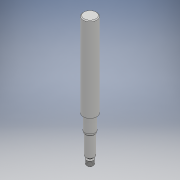
# Autodesk Inventor part: 도면1-2번
Saved by Autodesk Inventor 2018.3 (Build 223284000, 284)
## iProperties
Created: 2019-10-11
Part Number: 도면1-2번
Material: 일반
Document SubType Name: Modeling
Designer: MyTool
Density: 1 g/cm^3
Appearance: 기본값
Author: MyTool
Autodesk Inventor part; units mm, degrees
ref_plane "YZ Plane" through (0, 0, 0) normal (1, 0, 0) x (0, 1, 0)
ref_plane "XZ Plane" through (0, 0, 0) normal (0, 1, 0) x (-1, 0, 0)
ref_plane "XY Plane" through (0, 0, 0) normal (0, 0, 1) x (1, 0, 0)
sketch "스케치1" plane through (0, 0, 0) normal (1, 0, 0) x (0, 1, 0)
  line L0 (0, 0) -> (4, 0)
  line L1 (4, 0) -> (4, 10)
  line L2 (4, 10) -> (0, 10)
  line L3 (0, 10) -> (0, 0)
  line L4 (0, 10) -> (5, 10)
  line L5 (5, 10) -> (5, 33)
  line L6 (5, 33) -> (0, 33)
  line L7 (0, 33) -> (0, 10)
  line L8 (0, 33) -> (6, 33)
  line L9 (6, 33) -> (6, 53)
  line L10 (6, 53) -> (0, 53)
  line L11 (0, 53) -> (0, 33)
  line L12 (0, 53) -> (8, 53)
  line L13 (8, 53) -> (8, 153)
  line L14 (8, 153) -> (0, 153)
  line L15 (0, 153) -> (0, 53)
  dimension "d0" = 100
  dimension "d1" = 20
  dimension "d2" = 23
  dimension "d3" = 10
  dimension "d4" = 8
  dimension "d5" = 10
  dimension "d6" = 12
  dimension "d7" = 16
  constraints: 32 end point, 8 parallel, 4 horizontal, 4 perpendicular
  measures "d0" distance of L12.end L13.end
  measures "d1" distance of L8.end L9.end
  measures "d2" distance of L4.end L5.end
  measures "d3" distance of L0.end L1.end
  measures "d4" diameter of L1 L3
  measures "d5" diameter of L5 L7
  measures "d6" diameter of L9 L11
  measures "d7" diameter of L13 L15
revolve "회전1" add sketch "스케치1" angle 360 about axis through (0, 0, 33) along (0, 0, -1)
thread "스레드1" size "M8x1.25" class "6g" standard "ANSI Metric M Profile" full length
sketch "스케치2" plane through (0, 0, 0) normal (1, 0, 0) x (0, 1, 0)
  line L0 (6, 53) -> (6, 33) projected
  line L1 (-6, 33) -> (6, 33) projected
  line L2 (6, 33) -> (6, 34.5588)
  line L3 (6, 33) -> (5.1, 33)
  line L4 (5.1, 33) -> (6, 34.5588)
  line L5 (0, -30.6) -> (0, 183.6) projected
  point P0 (0, 0)
  dimension "d11" = 0.9
  dimension "d12" = 30
  constraints: 6 end point, 2 point on line
  measures "d11" distance of L0.end L3.end
  measures "d12" angle of L0 L4
revolve "회전2" cut sketch "스케치2" angle 360 about axis through (0, 0, -10) along (0, 0, 1)
fillet "모깎기1" radius 4 1 edges at (0, -6, 34.5588)
fillet "모깎기2" radius 1 1 edges at (0, -5.1, 33)
sketch "스케치3" plane through (0, 0, 0) normal (1, 0, 0) x (0, 1, 0)
  line L0 (5, 33) -> (5, 10) projected
  line L1 (5, 14) -> (3.2, 14)
  line L2 (3.2, 14) -> (3.2, 24)
  line L3 (3.2, 24) -> (5, 24)
  line L4 (5, 24) -> (5, 14)
  point P0 (0, 0)
  dimension "d16" = 1.8
  dimension "d17" = 10
  dimension "d18" = 4
  constraints: 8 end point, 2 parallel, 1 horizontal, 1 perpendicular, 1 point on line
  measures "d16" distance of L2.end L3.end
  measures "d17" distance between parallel lines of L3 L1
  measures "d18" distance from line of L1 L0.end
extrude "돌출1" cut sketch "스케치3" along normal mid plane 3
fillet "모깎기3" radius 1.5 4 edges at (1.5, 3.9848, 14) (-1.5, 3.9848, 14) (-1.5, 3.9848, 24) (1.5, 3.9848, 24)
chamfer "모따기1" distance 1 angle 45 2 edges at (0, -8, 153) (0, -4, 0)
sketch "스케치4" plane through (0, 0, 0) normal (1, 0, 0) x (0, 1, 0)
  line L0 (4, 10) -> (4, 6.25)
  line L1 (4, 6.25) -> (3, 8)
  line L2 (3, 8) -> (3, 10)
  line L3 (3, 10) -> (4, 10)
  line L4 (-5, 10) -> (5, 10) projected
  line L5 (0, -30.6) -> (0, 183.6) projected
  point P0 (0, 0)
  dimension "d25" = 1
  dimension "d26" = 2
  dimension "d27" = 3.75
  constraints: 8 end point, 1 collinear, 1 parallel, 1 vertical
  measures "d25" distance of L2.end L0.start
  measures "d26" distance of L1.end L2.end
  measures "d27" distance of L0.start L0.end
revolve "회전3" cut sketch "스케치4" angle 360 about axis through (0, 0, -10) along (0, 0, 1)
fillet "모깎기4" radius 0.6 2 edges at (0, -3, 8) (0, -3, 10)
